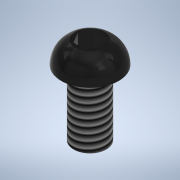
# Autodesk Inventor part: M2 6mm HEX
Saved by Autodesk Inventor 2022 (Build 260153000, 153)
## iProperties
Created: 2023-07-21
Part Number: M2 6mm HEX
Material: Типовые
Document SubType Name: Modeling
Designer: akapu
Density: 1 g/cm^3
Appearance: По умолчанию
Author: akapu
Autodesk Inventor part; units mm, degrees
ref_plane "YZ Plane" through (0, 0, 0) normal (1, 0, 0) x (0, 1, 0)
ref_plane "XZ Plane" through (0, 0, 0) normal (0, 1, 0) x (-1, 0, 0)
ref_plane "XY Plane" through (0, 0, 0) normal (0, 0, 1) x (1, 0, 0)
sketch "Эскиз1" plane through (0, 0, 0) normal (0, 1, 0) x (-1, 0, 0)
  circle A0 centre (0, 0) radius 1
  dimension "d0" = 2
  constraints: 1 centre point, 1 coincident
  measures "d0" diameter of A0
extrude "Выдавливание1" add sketch "Эскиз1" along normal blind 4
sketch "Эскиз2" plane through (0, 0, 0) normal (1, 0, 0) x (0, 1, 0)
  line L0 (4, -1) -> (4, 1) projected
  line L1 (4, 0) -> (5.3, 0)
  line L2 (4, 0) -> (4, -1.75)
  line L3 (5.3, 0) -> (5.3, -1.75)
  line L4 (5.3, -1.75) -> (4, -1.75)
  arc A0 (4, -1.75) -> (5.3, -0.875) centre (4, -0.3468) ccw
  point P0 (0, 0)
  dimension "d3" = 1.3
  dimension "d4" = 1.75
  constraints: 8 end point, 2 midpoint, 2 point on circle, 1 centre point, 1 horizontal, 1 point on line, 1 tangent, 1 vertical
  measures "d3" distance of L1.start L1.end
  measures "d4" distance of L1.start L2.end
revolve "Вращение1" add sketch "Эскиз2" angle 360 about axis through (0, 4, 0) along (0, 1, 0) contours L0 L1 L3 A0 L2
sketch "Эскиз3" plane through (0, 5.3, 0) normal (0, 1, 0) x (1, 0, 0)
  line L0 (0, 0) -> (0, 0.65)
  line L1 (0.3753, 0.65) -> (0.7506, 0)
  line L2 (0.7506, 0) -> (0.3753, -0.65)
  line L3 (0.3753, -0.65) -> (-0.3753, -0.65)
  line L4 (-0.3753, -0.65) -> (-0.7506, 0)
  line L5 (-0.7506, 0) -> (-0.3753, 0.65)
  line L6 (-0.3753, 0.65) -> (0.3753, 0.65)
  dimension "d6" = 0.65
  constraints: 14 end point, 1 coincident, 1 midpoint, 1 vertical, 13 other
  measures "d6" distance of L0.start L0.end
extrude "Выдавливание2" cut sketch "Эскиз3" against normal blind 1
thread "Резьба1" size "M2x0.4" class "6g" standard "ANSI Metric M Profile" length 19.85
